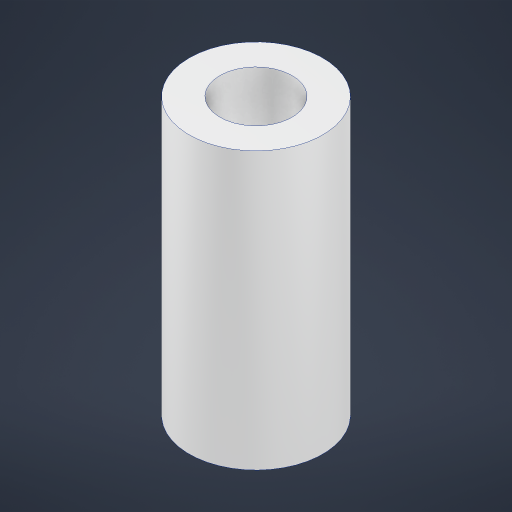
# Autodesk Inventor part: CORL_011_NEOStandoff
Saved by Autodesk Inventor 2024.2 (Build 282272000, 272)
## iProperties
Created: 2024-08-05
Part Number: CORL_011_NEOStandoff
Material: Aluminum 6061
Document SubType Name: Modeling
Designer: Bryan
Density: 2.7 g/cm^3
Appearance: Aluminum - Flat
Mass: 3.22398 g
Surface Area: 12.2541 cm^2
Volume: 1.19406 cm^3
Author: Bryan
Autodesk Inventor part; units mm, degrees
ref_plane "YZ Plane" through (0, 0, 0) normal (1, 0, 0) x (0, 1, 0)
ref_plane "XZ Plane" through (0, 0, 0) normal (0, 1, 0) x (-1, 0, 0)
ref_plane "XY Plane" through (0, 0, 0) normal (0, 0, 1) x (1, 0, 0)
sketch "Sketch1" plane through (0, 0, 0) normal (0, 1, 0) x (-1, 0, 0)
  circle A0 centre (0, 0) radius 25.4 construction
  circle A1 centre (0, 0) radius 30 construction
  circle A2 centre (25.4, 0) radius 2.4892
  circle A3 centre (25.4, 0) radius 4.6
  dimension "d0" = 50.8
  dimension "d1" = 60
  dimension "d2" = 4.9784
  constraints: 3 centre point, 3 coincident, 2 horizontal alignment, 1 tangent, 2 other
  measures "d1" diameter of A1
  measures "d2" diameter of A2
extrude "Extrusion1" add sketch "Sketch1" along normal blind 19.05
body "Solid1"
